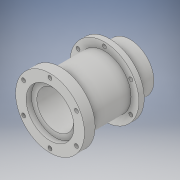
# Autodesk Inventor part: PostComb4_4
Saved by Autodesk Inventor 2017 (Build 210142000, 142)
## iProperties
Created: 2018-04-05
Part Number: PostComb4_4
Material: Generic
Document SubType Name: Modeling
Designer: Johnny
Density: 1 g/cm^3
Appearance: Default
Author: Johnny
Autodesk Inventor part; units mm, degrees
ref_plane "YZ Plane" through (0, 0, 0) normal (1, 0, 0) x (0, 1, 0)
ref_plane "XZ Plane" through (0, 0, 0) normal (0, 1, 0) x (-1, 0, 0)
ref_plane "XY Plane" through (0, 0, 0) normal (0, 0, 1) x (1, 0, 0)
sketch "Sketch1" plane through (0, 0, 0) normal (0, 0, 1) x (1, 0, 0)
  circle A0 centre (0, 0) radius 41.148
  dimension "d0" = 82.296
  constraints: 1 centre point, 1 coincident
  measures "d0" diameter of A0
extrude "Extrusion1" add sketch "Sketch1" against normal blind 95.504
sketch "Sketch2" plane through (0, 0, 0) normal (0, 0, 1) x (1, 0, 0)
  circle A0 centre (0, 0) radius 22.098
  dimension "d3" = 44.196
  constraints: 1 centre point, 1 coincident
  measures "d3" diameter of A0
extrude "Extrusion2" cut sketch "Sketch2" against normal blind 95.504
sketch "Sketch3" plane through (0, 0, -95.504) normal (0, 0, -1) x (-1, 0, 0)
  circle A0 centre (0, 0) radius 41.148
  circle A1 centre (0, 0) radius 28.575
  dimension "d6" = 57.15
  constraints: 2 centre point, 2 coincident
  measures "d6" diameter of A1
extrude "Extrusion3" cut sketch "Sketch3" against normal blind 24.13
sketch "Sketch4" plane through (0, 0, 0) normal (0, 0, 1) x (1, 0, 0)
  circle A0 centre (0, 0) radius 22.098
  circle A1 centre (0, 0) radius 28.575
  dimension "d9" = 57.15
  constraints: 2 centre point, 2 coincident
  measures "d9" diameter of A1
extrude "Extrusion4" cut sketch "Sketch4" against normal blind 6.35
sketch "Sketch5" plane through (0, 0, 0) normal (0, 0, 1) x (1, 0, 0)
  circle A0 centre (0, 0) radius 41.148
  circle A1 centre (0, 0) radius 31.75
  dimension "d12" = 63.5
  constraints: 2 centre point, 2 coincident
  measures "d12" diameter of A1
extrude "Extrusion5" cut sketch "Sketch5" against normal blind 65.024
sketch "Sketch6" plane through (0, 0, 0) normal (0, 0, 1) x (1, 0, 0)
  circle A0 centre (0, 0) radius 31.75
  circle A1 centre (0, 0) radius 41.148
  constraints: 2 centre point, 2 coincident
extrude "Extrusion6" add sketch "Sketch6" against normal blind 12.7
sketch "Sketch7" plane through (0, 0, 0) normal (0, 0, 1) x (1, 0, 0)
  circle A0 centre (0, 36.449) radius 2.3813
  circle A1 centre (-31.5658, 18.2245) radius 2.3813
  circle A2 centre (-31.5658, -18.2245) radius 2.3813
  circle A3 centre (0, -36.449) radius 2.3813
  circle A4 centre (31.5658, -18.2245) radius 2.3813
  circle A5 centre (31.5658, 18.2245) radius 2.3813
  point P0 (0, 0)
  dimension "d17" = 4.7625
  dimension "d20" = 360
  constraints: 6 centre point, 13 other
  measures "d17" diameter of A0
extrude "Extrusion7" cut sketch "Sketch7" against normal blind 152.4
body "Solid1"
